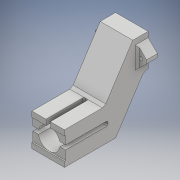
# Autodesk Inventor part: RescueKit-Pipev3
Saved by Autodesk Inventor 2018.3 (Build 223284000, 284)
## iProperties
Created: 2019-03-13
Part Number: RescueKit-Pipev3
Material: 一般
Document SubType Name: Modeling
Designer: shun2
Density: 1 g/cm^3
Appearance: 既定
Author: shun2
Autodesk Inventor part; units mm, degrees
ref_plane "YZ Plane" through (0, 0, 0) normal (1, 0, 0) x (0, 1, 0)
ref_plane "XZ Plane" through (0, 0, 0) normal (0, 1, 0) x (-1, 0, 0)
ref_plane "XY Plane" through (0, 0, 0) normal (0, 0, 1) x (1, 0, 0)
sketch "スケッチ1" plane through (0, 0, 0) normal (1, 0, 0) x (0, 1, 0)
  line L0 (-10, 0) -> (18.2843, 0) construction
  line L1 (-10, 0) -> (34.366, 0) construction
  line L2 (-75, -65) -> (-27.8868, -65)
  line L3 (-38.094, -35) -> (-75, -35)
  line L4 (-75, -35) -> (-75, -65)
  line L5 (0, 5) -> (-12.1177, 5)
  line L6 (-15, 5) -> (31.188, 5) construction
  line L7 (-25, -60) -> (-19.2265, -60) construction
  line L8 (-1.9104, -25) -> (0, -25)
  line L9 (0, 5) -> (2, 5)
  line L10 (2, 5) -> (2, -25)
  line L11 (2, -25) -> (0, -25)
  line L12 (-27.8868, -65) -> (-1.9104, -25)
  line L13 (-27.8868, -65) -> (19.8078, -65) construction
  line L14 (-38.094, -35) -> (-12.1177, 5)
  line L15 (-10.7143, -35) -> (9.6005, -35) construction
  point P0 (0, 0)
  dimension "d49" = 2
  dimension "d50" = 57
  constraints: 32 end point, 9 horizontal, 3 parallel, 1 equal length, 1 perpendicular, 1 point on line
  measures "d49" distance of L10.end L8.end
  measures "d50" angle of L13 L12
extrude "押し出し1" add sketch "スケッチ1" along normal blind 20
sketch "スケッチ2" plane through (20, 0, 0) normal (1, 0, 0) x (0, 0, -1)
  line L0 (65, -75) -> (65, -27.8868) projected
  line L1 (65, -27.8868) -> (25, -1.9104) projected
  line L2 (25, -1.9104) -> (25, 2) projected
  line L3 (25, 2) -> (-5, 2) projected
  line L4 (-5, 2) -> (-5, -12.1177) projected
  line L5 (-5, -12.1177) -> (35, -38.094) projected
  line L6 (35, -38.094) -> (35, -75) projected
  line L7 (35, -75) -> (65, -75) projected
  line L8 (65, -75) -> (65, -27.8868) projected
  line L9 (65, -27.8868) -> (25, -1.9104) projected
  line L10 (25, -1.9104) -> (25, 2) projected
  line L11 (25, 2) -> (-5, 2) projected
  line L12 (-5, 2) -> (-5, -12.1177) projected
  line L13 (-5, -12.1177) -> (35, -38.094) projected
  line L14 (35, -38.094) -> (35, -75) projected
  line L15 (35, -75) -> (65, -75) projected
  line L16 (35, -75) -> (65, -75) projected
  line L17 (40, -75) -> (60, -75)
  line L18 (60, -75) -> (60, -29.4241)
  line L19 (40, -35) -> (40, -75)
  line L20 (40, -35) -> (0, -9.0237)
  line L21 (60, -29.4241) -> (20, -3.4478)
  line L22 (60, -29.4241) -> (112.0643, -29.4241) construction
  line L23 (0, 2) -> (20, 2)
  line L24 (20, 2) -> (20, -3.4478)
  line L25 (0, -9.0237) -> (0, 2)
  dimension "d53" = 147
  constraints: 18 end point, 3 horizontal, 2 parallel, 2 perpendicular, 1 point on line
  measures "d53" angle of L22 L21
extrude "押し出し2" cut sketch "スケッチ2" against normal blind 20 contours L7 L19 L20 L25 L3 L24 L21 L18
sketch "スケッチ3" plane through (20, 0, 0) normal (1, 0, 0) x (0, 0, -1)
  line L0 (35, -75) -> (40, -75) projected
  line L1 (35, -75) -> (40, -75) projected
  line L2 (0, 2) -> (-5, 2) projected
  line L3 (0, 2) -> (-5, 2) projected
  line L4 (20, 2) -> (20, -3.4478) projected
  line L5 (0, -9.0237) -> (0, 2) projected
  line L6 (40, -35) -> (0, -9.0237) projected
  line L7 (40, -75) -> (40, -35) projected
  line L8 (60, -29.4241) -> (60, -75) projected
  line L9 (20, -3.4478) -> (60, -29.4241) projected
  line L10 (20, 2) -> (20, -3.4478) projected
  line L11 (0, -9.0237) -> (0, 2) projected
  line L12 (40, -35) -> (0, -9.0237) projected
  line L13 (40, -75) -> (40, -35) projected
  line L14 (60, -29.4241) -> (60, -75) projected
  line L15 (20, -3.4478) -> (60, -29.4241) projected
  line L16 (-5, 2) -> (-5, -12.1177) projected
  line L17 (-5, -12.1177) -> (35, -38.094) projected
  line L18 (35, -38.094) -> (35, -75) projected
  line L19 (60, -75) -> (65, -75) projected
  line L20 (65, -75) -> (65, -27.8868) projected
  line L21 (65, -27.8868) -> (25, -1.9104) projected
  line L22 (25, -1.9104) -> (25, 2) projected
  line L23 (25, 2) -> (20, 2) projected
  line L24 (-5, 2) -> (-5, -12.1177) projected
  line L25 (-5, -12.1177) -> (35, -38.094) projected
  line L26 (35, -38.094) -> (35, -75) projected
  line L27 (60, -75) -> (65, -75) projected
  line L28 (65, -75) -> (65, -27.8868) projected
  line L29 (65, -27.8868) -> (25, -1.9104) projected
  line L30 (25, -1.9104) -> (25, 2) projected
  line L31 (25, 2) -> (20, 2) projected
  line L32 (-5, 2) -> (25, 2)
  line L33 (35, -75) -> (40, -75) projected
  line L34 (35, -75) -> (65, -75)
  line L35 (65, -75) -> (65, -27.8868) projected
  line L36 (65, -27.8868) -> (25, -1.9104) projected
  line L37 (65, -27.8868) -> (25, -1.9104)
  line L38 (25, -1.9104) -> (25, 2)
  line L39 (-5, 2) -> (-5, -12.1177) projected
  line L40 (-5, 2) -> (-5, -12.1177)
  line L41 (-5, -12.1177) -> (35, -38.094)
  line L42 (35, -75) -> (35, -38.094)
  line L43 (65, -75) -> (65, -27.8868)
  constraints: 16 end point, 4 collinear, 1 horizontal, 1 parallel, 1 perpendicular, 1 vertical
extrude "押し出し3" add sketch "スケッチ3" along normal blind 5
sketch "スケッチ4" plane through (0, 0, 0) normal (-1, 0, 0) x (0, 0, 1)
  line L0 (-60, -75) -> (-65, -75) projected
  line L1 (-60, -75) -> (-65, -75) projected
  line L2 (-25, 2) -> (-20, 2) projected
  line L3 (-25, 2) -> (-20, 2) projected
  line L4 (-20, -3.4478) -> (-20, 2) projected
  line L5 (-60, -29.4241) -> (-20, -3.4478) projected
  line L6 (-60, -75) -> (-60, -29.4241) projected
  line L7 (-40, -35) -> (-40, -75) projected
  line L8 (0, -9.0237) -> (-40, -35) projected
  line L9 (0, 2) -> (0, -9.0237) projected
  line L10 (-20, -3.4478) -> (-20, 2) projected
  line L11 (-60, -29.4241) -> (-20, -3.4478) projected
  line L12 (-60, -75) -> (-60, -29.4241) projected
  line L13 (-40, -35) -> (-40, -75) projected
  line L14 (0, -9.0237) -> (-40, -35) projected
  line L15 (0, 2) -> (0, -9.0237) projected
  line L16 (-35, -75) -> (-40, -75) projected
  line L17 (-35, -38.094) -> (-35, -75) projected
  line L18 (5, -12.1177) -> (-35, -38.094) projected
  line L19 (5, 2) -> (5, -12.1177) projected
  line L20 (0, 2) -> (5, 2) projected
  line L21 (-25, -1.9104) -> (-25, 2) projected
  line L22 (-65, -27.8868) -> (-25, -1.9104) projected
  line L23 (-65, -75) -> (-65, -27.8868) projected
  line L24 (-35, -75) -> (-40, -75) projected
  line L25 (-35, -38.094) -> (-35, -75) projected
  line L26 (5, -12.1177) -> (-35, -38.094) projected
  line L27 (5, 2) -> (5, -12.1177) projected
  line L28 (0, 2) -> (5, 2) projected
  line L29 (-25, -1.9104) -> (-25, 2) projected
  line L30 (-65, -27.8868) -> (-25, -1.9104) projected
  line L31 (-65, -75) -> (-65, -27.8868) projected
  line L32 (-25, 2) -> (-20, 2) projected
  line L33 (-25, 2) -> (5, 2)
  line L34 (5, 2) -> (5, -12.1177) projected
  line L35 (5, 2) -> (5, -12.1177)
  line L36 (5, -12.1177) -> (-35, -38.094) projected
  line L37 (-35, -38.094) -> (5, -12.1177)
  line L38 (-25, -1.9104) -> (-25, 2) projected
  line L39 (-25, 2) -> (-25, -1.9104)
  line L40 (-65, -27.8868) -> (-25, -1.9104) projected
  line L41 (-25, -1.9104) -> (-65, -27.8868)
  line L42 (-65, -75) -> (-65, -27.8868) projected
  line L43 (-65, -27.8868) -> (-65, -75)
  line L44 (-65, -75) -> (-35, -75)
  line L45 (-35, -38.094) -> (-35, -75)
  point P0 (-25, 0)
  constraints: 16 end point, 5 collinear, 1 parallel, 1 perpendicular, 1 vertical
extrude "押し出し4" add sketch "スケッチ4" along normal blind 5
sketch "スケッチ5" plane through (25, 0, 0) normal (1, 0, 0) x (0, 0, -1)
  line L0 (-5, -12.1177) -> (35, -38.094) projected
  line L1 (35, -38.094) -> (35, -75) projected
  line L2 (35, -75) -> (65, -75) projected
  line L3 (65, -75) -> (65, -27.8868) projected
  line L4 (65, -27.8868) -> (25, -1.9104) projected
  line L5 (25, -1.9104) -> (25, 2) projected
  line L6 (25, 2) -> (-5, 2) projected
  line L7 (-5, 2) -> (-5, -12.1177) projected
  point P0 (0, 0)
chamfer "面取り1" distance 2 angle 45 2 edges at (10, -38.094, -35) (10, -1.9104, -25)
sketch "スケッチ6" plane through (25, -75, -65) normal (0, -1, 0) x (1, 0, 0)
  circle A0 centre (-15, 15) radius 10
  line L0 (-5, 5) -> (-25, 5) projected
  line L1 (-25, 25) -> (-5, 25) projected
  line L2 (0, 0) -> (-30, 0) projected
  line L3 (-30, 30) -> (0, 30) projected
  line L4 (0, 30) -> (0, 0) projected
  line L5 (-5, 25) -> (-5, 5) projected
  line L6 (-30, 0) -> (-30, 30) projected
  line L7 (-25, 5) -> (-25, 25) projected
  point P0 (-25, 65)
  dimension "d31" = 20
  constraints: 1 centre point
  measures "d31" diameter of A0
extrude "押し出し5" add sketch "スケッチ6" against normal blind 40 contours L5 L0 A0 | A0 L1 L5 | A0 L7 L1 | L0 L7 A0 | L2 L6 L3 L4
sketch "スケッチ8" plane through (25, -75, -65) normal (0, -1, 0) x (1, 0, 0)
  line L0 (0, 25) -> (-30, 25)
  line L1 (-30, 25) -> (-30, 5)
  line L2 (-30, 5) -> (0, 5)
  line L3 (0, 5) -> (0, 25)
  point P0 (-25, 65)
  constraints: 8 end point, 2 parallel, 1 horizontal, 1 perpendicular
extrude "押し出し7" cut sketch "スケッチ8" against normal blind 1
sketch "スケッチ9" plane through (25, 2, 5) normal (0, 1, 0) x (1, 0, 0)
  circle A0 centre (-33.6, 15) radius 1.6
  line L0 (-30, 38.3227) -> (-30, 0) projected
  line L1 (-30, 5) -> (-38.5697, 13.4)
  line L2 (-15, 8.2441) -> (-15, 19.5683)
  line L3 (-30, 25) -> (-38.5697, 16.6)
  line L4 (-38.5697, 16.6) -> (-38.5697, 13.4)
  line L5 (-30, 5) -> (-30, 25)
  circle A1 centre (3.6, 15) radius 1.6
  line L6 (0, 5) -> (8.5697, 13.4)
  line L7 (0, 25) -> (8.5697, 16.6)
  line L8 (8.5697, 16.6) -> (8.5697, 13.4)
  line L9 (0, 5) -> (0, 25)
  point P0 (-25, 5)
  point P1 (-15, 15)
  dimension "d55" = 3.2
  dimension "d57" = 12
  dimension "d58" = 12
  constraints: 18 end point, 5 symmetric about line, 2 centre point, 2 point on line, 2 vertical, 1 collinear, 1 other
  measures "d55" diameter of A0
  measures "d57" distance of L1.start L1.end
  measures "d58" distance of L3.start L3.end
extrude "押し出し8" add sketch "スケッチ9" against normal blind 10
chamfer "面取り4" distance 2 angle 45 2 edges at (-5, -8, -10) (25, -8, -10)
sketch "スケッチ10" plane through (25, 0, 0) normal (1, 0, 0) x (0, 0, -1)
  line L0 (60, -74) -> (40, -74) projected
  line L1 (51.5, -35) -> (47.5, -35)
  line L2 (47.5, -35) -> (47.5, -74)
  line L3 (47.5, -74) -> (51.5, -74)
  line L4 (51.5, -74) -> (51.5, -35)
  line L5 (51.5, -35) -> (47.5, -74) construction
  line L6 (47.5, -35) -> (51.5, -74) construction
  point P0 (0, 0)
  point P1 (50, -74)
  point P2 (49.5, -54.5)
  dimension "d64" = 4
  constraints: 12 end point, 3 midpoint, 2 parallel, 1 horizontal, 1 perpendicular, 1 point on line
  measures "d64" distance of L3.end L2.end
extrude "押し出し9" cut sketch "スケッチ10" against normal blind 100
sketch "スケッチ11" plane through (-5, -75, -35) normal (0, 0, 1) x (1, 0, 0)
  line L0 (0, 0) -> (30, 0) projected
  line L1 (13, 39) -> (17, 39)
  line L2 (17, 39) -> (17, 0)
  line L3 (17, 0) -> (13, 0)
  line L4 (13, 0) -> (13, 39)
  line L5 (13, 39) -> (17, 0) construction
  line L6 (17, 39) -> (13, 0) construction
  line L7 (0, 34.906) -> (30, 34.906) projected
  line L8 (17, 34.906) -> (13, 34.906)
  point P0 (5, 75)
  point P1 (15, 19.5)
  dimension "d67" = 4
  constraints: 14 end point, 5 point on line, 2 midpoint, 2 parallel, 1 horizontal, 1 perpendicular
  measures "d67" distance of L2.end L3.end
extrude "押し出し10" cut sketch "スケッチ11" against normal blind 8 contours L4 L7 L2 L0
chamfer "面取り5" distance 1 angle 45 6 edges at (8, -40.094, -37.601) (12, -40.094, -37.601) (22.5, -35, -51.5) (22.5, -35, -47.5) (-2.5, -35, -51.5) (-2.5, -35, -47.5)
